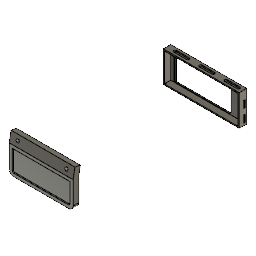
GPU mount (Autodesk Fusion 360 design; units mm, degrees)
Autodesk Fusion 360 part; units mm, degrees
sketch "imac body" plane through (0, 0, 0) normal (0, 0, 1) x (1, 0, 0)
  line L0 (-150, -55) -> (150, -55)
  line L1 (150, -55) -> (150, 150)
  line L2 (20, 280) -> (-20, 280)
  line L3 (-150, 150) -> (-150, -55)
  line L4 (0, 280) -> (0, -55) construction
  line L5 (0, 0) -> (150, 0) construction
  arc A0 (-20, 280) -> (-150, 150) centre (-20, 150) ccw
  arc A1 (150, 150) -> (20, 280) centre (20, 150) ccw
  line L6 (150, 0) -> (-150, 0)
  line L7 (-93.6888, 60) -> (93.6888, 60)
  line L8 (93.6888, 60) -> (93.6888, 40)
  line L9 (93.6888, 40) -> (-93.6888, 40)
  line L10 (-93.6888, 40) -> (-93.6888, 60)
  dimension "d1" = 280
  dimension "d2" = 55
  dimension "d3" = 300
  dimension "d4" = 130
  dimension "d7" = 40
  dimension "d8" = 20
  constraint horizontal L0
  constraint vertical L1
  constraint horizontal L2
  constraint vertical L3
  constraint midpoint L0 L4.end
  constraint coincident L5.start L4
  constraint coincident L5.start origin
  constraint coincident L1 L5.end
  constraint perpendicular L1 L5
  constraint coincident L2 L4.start
  constraint tangent L2 A0
  constraint tangent L3 A0
  constraint tangent L1 A1
  constraint tangent L2 A1
  constraint equal A0 A1
  constraint coincident L3 L6.end
  constraint perpendicular L3 L6
  constraint horizontal L7
  constraint vertical L8
  constraint horizontal L9
  constraint vertical L10
  measures "d1" distance of L2 L5
  measures "d2" distance of L0 L5 L3.end
  measures "d3" distance of L1 L3
  measures "d4" radius of A0
  measures "d7" distance of L6 L9
  measures "d8" distance of L7 L9
  measures "d62" distance of L0.start
  measures "d83" distance of L0.start
extrude "Extrude1" add sketch "imac body" along normal blind 2 contours L1 L2 L3 A0 A1 L6 | L7 L8 L9 L10 makes body 1
extrude "Extrude2" add sketch "imac body" against normal blind 5 contours L7 L8 L9 L10 bodies 1
ref_plane "WorkPlane1" through (0, 0, 0) normal (0, 0.173648, 0.984808) x (-1, 0, 0)
sketch "imac body bend" plane through (0, 0, 0) normal (0, 0.173648, 0.984808) x (-1, 0, 0)
  line L0 (-150, 0) -> (150, 0)
  line L1 (-150, 0) -> (150, 0)
  line L2 (150, 0) -> (150, 55)
  line L3 (150, 55) -> (-150, 55)
  line L4 (-150, 55) -> (-150, 0)
  dimension "d32" = 55
  constraint horizontal L1
  constraint vertical L2
  constraint horizontal L3
  constraint vertical L4
  constraint coincident L0.start L1.start
  measures "d32" distance of L0.start L3.end
extrude "Extrude3" add sketch "imac body bend" along normal blind 2 bodies 1
sketch "gpu body" plane through (0, 0, 0) normal (0, 0, 1) x (1, 0, 0)
  line L0 (47.5, 132.5) -> (-47.5, 132.5)
  line L1 (-47.5, 132.5) -> (-47.5, -132.5)
  line L2 (-47.5, -132.5) -> (47.5, -132.5)
  line L3 (47.5, -132.5) -> (47.5, 132.5)
  line L4 (47.5, 132.5) -> (-47.5, -132.5) construction
  line L5 (-47.5, 132.5) -> (47.5, -132.5) construction
  line L6 (0, 132.5) -> (0, -132.5) construction
  circle A0 centre (0, -59.5) radius 32.5
  line L7 (-47.5, 132.5) -> (47.5, 132.5)
  line L8 (47.5, 132.5) -> (47.5, 136.5)
  line L9 (47.5, 136.5) -> (-47.5, 136.5)
  line L10 (-47.5, 136.5) -> (-47.5, 132.5)
  line L11 (-44.5, 136.5) -> (-42.5, 136.5)
  line L12 (-42.5, 136.5) -> (-42.5, 148.5)
  line L13 (-42.5, 148.5) -> (-44.5, 148.5)
  line L14 (-44.5, 148.5) -> (-44.5, 136.5)
  line L15 (-44.5, 136.5) -> (-44.5, 132.5)
  dimension "d14" = 265
  dimension "d15" = 95
  dimension "d18" = 65
  dimension "d19" = 73
  dimension "d20" = 4
  dimension "d21" = 2
  dimension "d22" = 12
  dimension "d23" = 3
  constraint perpendicular L0 L1
  constraint parallel L0 L2
  constraint parallel L1 L3
  constraint horizontal L0
  constraint coincident L4 origin
  constraint coincident L5 origin
  constraint midpoint L0 L6.start
  constraint midpoint L2 L6.end
  constraint coincident L6 A0.centre
  constraint horizontal L7
  constraint vertical L8
  constraint horizontal L9
  constraint vertical L10
  constraint horizontal L11
  constraint vertical L12
  constraint horizontal L13
  constraint vertical L14
  constraint coincident L9 L11.start
  constraint coincident L7 L15.end
  constraint perpendicular L7 L15
  measures "d14" distance of L0.end L1.end
  measures "d15" distance of L1.end L2.end
  measures "d18" diameter of A0
  measures "d19" distance of L6.end A0.centre
  measures "d20" distance of L7 L9
  measures "d21" distance of L12 L14
  measures "d22" distance of L9 L13
  measures "d23" distance of L9.end L11.start
extrude "Extrude4" add sketch "gpu body" against normal blind 37 separate body contours L0 L1 L2 L3 L7 | L0 L7 L8 L9 L11 L15 | L9 L11 L12 L13 L14 | A0 makes body 2
extrude "Extrude5" cut sketch "gpu body" along normal blind 3 from surface at -37 contours A0 bodies 2
sketch "gpu psu connector" plane through (-47.5, 0, 0) normal (-1, 0, 0) x (0, -1, 0)
  line L0 (132.5, 0) -> (-132.5, 0)
  line L1 (-132.5, 0) -> (-132.5, -37)
  line L2 (-132.5, -37) -> (132.5, -37)
  line L3 (132.5, -37) -> (132.5, 0)
  line L4 (122.5, 0) -> (80.5, 0)
  line L5 (80.5, 0) -> (80.5, -20)
  line L6 (80.5, -20) -> (122.5, -20)
  line L7 (122.5, -20) -> (122.5, 0)
  dimension "d27" = 10
  dimension "d28" = 42
  dimension "d29" = 20
  constraint horizontal L4
  constraint vertical L5
  constraint horizontal L6
  constraint vertical L7
  constraint coincident L0 L4.start
  measures "d27" distance of L3 L7
  measures "d28" distance of L5 L7
  measures "d29" distance of L4 L6
extrude "Extrude6" add sketch "gpu psu connector" along normal blind 10 contours L0 L4 L5 L6 L7 bodies 2
move_body "Move5" bodies 2 to x (1, 0, 0) y (0, 1, 0) z (0, 0, 1) at (0, 63, -10)
sketch "gpu front connector" plane through (47.5, 0, 0) normal (1, 0, 0) x (0, 1, 0)
  line L0 (199.5, -47) -> (199.5, -10)
  line L1 (199.5, -10) -> (-69.5, -10)
  line L2 (-69.5, -10) -> (-69.5, -47)
  line L3 (197.0366, -14.7221) -> (198.5366, -14.7221)
  line L4 (198.5366, -14.7221) -> (198.5366, -24.7221)
  line L5 (198.5366, -24.7221) -> (197.0366, -24.7221)
  line L6 (197.0366, -24.7221) -> (197.0366, -14.7221)
  line L7 (197.0366, -34.7221) -> (198.5366, -34.7221)
  line L8 (198.5366, -34.7221) -> (198.5366, -44.7221)
  line L9 (198.5366, -44.7221) -> (197.0366, -44.7221)
  line L10 (197.0366, -44.7221) -> (197.0366, -34.7221)
  circle A0 centre (203.3196, -12.8419) radius 2.25
  circle A1 centre (203.3196, -28.3419) radius 2.25
  line L11 (-69.5, -47) -> (199.5, -47)
  line L12 (199.5, -47) -> (196.0366, -47)
  line L13 (196.0366, -47) -> (196.0366, -10)
  line L14 (196.0366, -10) -> (199.5, -10)
  line L15 (199.5, -10) -> (199.5, -47)
  line L16 (199.0366, -25.2221) -> (196.5366, -25.2221)
  line L17 (196.5366, -25.2221) -> (196.5366, -14.2221)
  line L18 (196.5366, -14.2221) -> (199.0366, -14.2221)
  line L19 (199.0366, -14.2221) -> (199.0366, -25.2221)
  line L20 (199.0366, -45.2221) -> (196.5366, -45.2221)
  line L21 (196.5366, -45.2221) -> (196.5366, -34.2221)
  line L22 (196.5366, -34.2221) -> (199.0366, -34.2221)
  line L23 (199.0366, -34.2221) -> (199.0366, -45.2221)
  dimension "d61" = 1.5
  dimension "d62" = 10
  dimension "d63" = 1.5
  dimension "d64" = 10
  dimension "d65" = 10
  dimension "d69" = 4.5
  dimension "d70" = 4.5
  dimension "d71" = 15.5
  dimension "d83" = 1
  dimension "d84" = -0.5
  dimension "d85" = -0.5
  constraint horizontal L3
  constraint vertical L4
  constraint horizontal L5
  constraint vertical L6
  constraint horizontal L7
  constraint vertical L8
  constraint horizontal L9
  constraint vertical L10
  constraint horizontal L12
  constraint vertical L13
  constraint horizontal L14
  constraint vertical L15
  constraint coincident L1 L13.end
  constraint coincident L0.start L11.end
  constraint collinear L17 L21
  measures "d61" distance of L3.start L3.end
  measures "d62" distance of L3.start L5.end
  measures "d63" distance of L7.start L7.end
  measures "d64" distance of L7.start L9.end
  measures "d65" distance of L5 L7
  measures "d69" diameter of A0
  measures "d70" diameter of A1
  measures "d71" distance of A0.centre A1.centre
  measures "d83" distance of L6 L13
extrude "Extrude13" add sketch "gpu front connector" along normal blind 29 contours L3 L4 L5 L6 | L7 L8 L9 L10 bodies 2
extrude "Extrude14" cut sketch "gpu front connector" against normal blind 100 contours A0 | A1 bodies 2
fillet "Fillet2" radius 4 2 edges at (-47.5, 63, -47) (47.5, 65, -47) on bodies 2
sketch "gpu front mount" plane through (0, 199.5, 0) normal (0, 1, 0) x (-1, 0, 0)
  arc A0 (-47.5, -43) -> (-43.5, -47) centre (-43.5, -43) ccw
  line L0 (-43.5, -47) -> (42.5, -47)
  line L1 (42.5, -47) -> (42.5, -10)
  line L2 (42.5, -10) -> (-47.5, -10)
  line L3 (-47.5, -10) -> (-47.5, -43)
  line L4 (44.5, -10) -> (44.5, -46.873)
  line L5 (47.5, -10) -> (47.5, -43)
  line L6 (-47.5, -14.7221) -> (-76.5, -14.7221)
  line L7 (-76.5, -24.7221) -> (-76.5, -14.7221)
  line L8 (-47.5, -24.7221) -> (-76.5, -24.7221)
  line L9 (-47.5, -34.7221) -> (-76.5, -34.7221)
  line L10 (-76.5, -44.7221) -> (-76.5, -34.7221)
  line L11 (-76.5, -44.7221) -> (-47.1103, -44.7221)
  line L12 (-43.5, -49) -> (42.5, -49) construction
  line L13 (-67.5, -49) -> (50.5, -49)
  line L14 (50.5, -49) -> (50.5, 0)
  line L15 (-67.5, 0) -> (-67.5, -49)
  arc A1 (-46.5, -43) -> (-43.5, -46) centre (-43.5, -43) ccw
  line L16 (-43.5, -46) -> (41.5, -46)
  line L17 (41.5, -46) -> (41.5, -11)
  line L18 (41.5, -11) -> (-46.5, -11)
  line L19 (-46.5, -11) -> (-46.5, -43)
  line L20 (150, 0) -> (20, 0)
  line L21 (-20, 0) -> (20, 0)
  line L22 (-20, 0) -> (-150, 0)
  line L23 (-43.5, -47) -> (-67.5, -47)
  arc A2 (43.5, -47) -> (44.5, -46.873) centre (43.5, -43) ccw
  line L24 (44.5, -46.873) -> (44.5, -10)
  line L25 (44.5, -10) -> (42.5, -10)
  line L26 (42.5, -10) -> (42.5, -47)
  line L27 (42.5, -47) -> (43.5, -47)
  line L28 (43.5, -47) -> (50.5, -47)
  line L29 (48.5, 0) -> (48.5, -47)
  dimension "d75" = 2
  dimension "d76" = -1
  dimension "d81" = 6
  dimension "d82" = 112
  dimension "d99" = 2
  constraint horizontal L13
  constraint vertical L14
  constraint vertical L15
  constraint coincident L12.start L13
  constraint coincident L15.start L22
  constraint coincident L14.end L20
  constraint coincident A0.end L0.start
  constraint tangent A0 L23
  constraint coincident L15 L23.end
  constraint coincident A2.start L27.end
  constraint coincident L14 L28.end
  constraint tangent A2 L28
  constraint coincident L20 L29.start
  constraint coincident L28 L29.end
  constraint perpendicular L28 L29
  measures "d81" distance of L4 L14
  measures "d82" distance of L4 L15
  measures "d99" distance of L14 L29
extrude "Extrude15" add sketch "gpu front mount" along normal blind 2 separate body contours A0 L0 L1 L2 L3 L26 | A0 L3 L9 L11 L15 | A0 L11 L15 L23 | L3 L8 L9 L15 | L0 L13 L14 L15 L23 L27 L28 | L3 L6 L8 L15 | L2 L3 L4 L6 L15 L20 L21 L22 A2 L24 L25 L28 L29 | L14 L20 L28 L29 makes body 3
extrude "Extrude17" add sketch "gpu front mount" against normal blind 10 contours L0 L13 L14 L15 L23 L27 L28 | L14 L20 L28 L29 bodies 3
sketch "gpu front mount side" plane through (47.5, 0, 0) normal (1, 0, 0) x (0, 1, 0)
  line L0 (198.5366, -43) -> (199.5, -43)
  line L1 (199.5, -10) -> (-69.5, -10)
  line L2 (-69.5, -10) -> (-69.5, -43)
  line L3 (-69.5, -43) -> (197.0366, -43)
  line L4 (197.0366, -43) -> (197.0366, -34.7221)
  line L5 (197.0366, -34.7221) -> (198.5366, -34.7221)
  line L6 (198.5366, -34.7221) -> (198.5366, -43)
  line L7 (197.0366, -24.7221) -> (197.0366, -14.7221)
  line L8 (197.0366, -14.7221) -> (198.5366, -14.7221)
  line L9 (198.5366, -14.7221) -> (198.5366, -24.7221)
  line L10 (198.5366, -24.7221) -> (197.0366, -24.7221)
  line L11 (196.5366, -34.2221) -> (199.0366, -34.2221)
  line L12 (196.5366, -45.2221) -> (196.5366, -34.2221)
  line L13 (199.0366, -34.2221) -> (199.0366, -45.2221)
  line L14 (199.0366, -45.2221) -> (196.5366, -45.2221)
  line L15 (199.0366, -25.2221) -> (196.5366, -25.2221)
  line L16 (196.5366, -25.2221) -> (196.5366, -14.2221)
  line L17 (199.0366, -14.2221) -> (199.0366, -25.2221)
  line L18 (196.5366, -14.2221) -> (199.0366, -14.2221)
  line L19 (199.5, 0) -> (199.5, -47)
  line L20 (189.5, -49) -> (201.5, -49)
  line L21 (201.5, -49) -> (201.5, 0)
  line L22 (201.5, 0) -> (199.5, 0)
  line L23 (199.5, -47) -> (189.5, -47)
  line L24 (189.5, -47) -> (189.5, 0)
  line L25 (189.5, 0) -> (199.5, 0)
  line L26 (199.5, 0) -> (199.5, -47)
  line L27 (199.5, -47) -> (189.5, -47)
  line L28 (189.5, -47) -> (189.5, -49)
  line L29 (199.5, -43) -> (199.5, -10)
  dimension "d86" = 10
  constraint horizontal L23
  constraint vertical L24
  constraint horizontal L25
  constraint vertical L26
  constraint coincident L19.end L23.start
  constraint coincident L19.start L22.end
  measures "d86" distance of L19.end L23.end
extrude "Extrude16" add sketch "gpu front mount side" along normal blind 2 from surface at 20 contours L0 L1 L3 L11 L12 L13 L19 L24 L26 L29 | L0 L3 L12 L13 L14 L19 L23 L24 L26 L27 | L19 L20 L21 L22 L23 L26 L27 L28 L29 | L1 L19 L24 L25 L26 bodies 3
sketch "gpu front mount top" plane through (0, 0, 0) normal (0, 0, -1) x (1, 0, 0)
  line L0 (93.6888, -40) -> (93.6888, -60)
  line L1 (93.6888, -60) -> (-93.6888, -60)
  line L2 (-93.6888, -60) -> (-93.6888, -40)
  line L3 (-93.6888, -40) -> (93.6888, -40)
  arc A0 (20, -280) -> (150, -150) centre (20, -150) ccw
  line L4 (150, -150) -> (150, 0)
  line L5 (150, 0) -> (-150, 0)
  line L6 (-150, 0) -> (-150, -150)
  arc A1 (-150, -150) -> (-20, -280) centre (-20, -150) ccw
  line L7 (-20, -280) -> (20, -280)
  line L8 (-50.5, -189.5) -> (-50.5, -201.5)
  line L9 (-50.5, -201.5) -> (69.5, -201.5)
  line L10 (69.5, -201.5) -> (69.5, -189.5)
  line L11 (69.5, -189.5) -> (-50.5, -189.5)
  circle A2 centre (-37.581, -195.5) radius 2.25
  circle A3 centre (-17.581, -195.5) radius 2.25
  circle A4 centre (2.419, -195.5) radius 2.25
  circle A5 centre (22.419, -195.5) radius 2.25
  circle A6 centre (42.419, -195.5) radius 2.25
  circle A7 centre (62.419, -195.5) radius 2.25
  line L12 (-37.581, -193.25) -> (-17.581, -193.25)
  line L13 (-17.581, -197.75) -> (-37.581, -197.75)
  line L14 (2.419, -193.25) -> (22.419, -193.25)
  line L15 (22.419, -197.75) -> (2.419, -197.75)
  line L16 (42.419, -193.25) -> (62.419, -193.25)
  line L17 (62.419, -197.75) -> (42.419, -197.75)
  dimension "d92" = 4.5
  dimension "d95" = 100
  dimension "d96" = 0
  constraint coincident A2 L12.start
  constraint coincident A3 L12.end
  constraint tangent A3 L12
  constraint perpendicular L8 L12
  constraint coincident A3 L13.start
  constraint coincident A2 L13.end
  constraint tangent A2 L13
  constraint perpendicular L8 L13
  constraint coincident A4 L14.start
  constraint coincident A5 L14.end
  constraint tangent A5 L14
  constraint parallel L13 L14
  constraint coincident A5 L15.start
  constraint coincident A4 L15.end
  constraint tangent A4 L15
  constraint parallel L14 L15
  constraint coincident A6 L16.start
  constraint coincident A7 L16.end
  constraint tangent A7 L16
  constraint parallel L15 L16
  constraint coincident A7 L17.start
  constraint coincident A6 L17.end
  constraint tangent A6 L17
  constraint parallel L16 L17
  measures "d92" diameter of A2
extrude "Extrude18" add sketch "gpu front mount top" along normal blind 2 contours L8 L9 L10 L11 bodies 3
sketch "gpu back back side" plane through (0, -69.5, 0) normal (0, -1, 0) x (1, 0, 0)
  arc A0 (43.5, -47) -> (47.5, -43) centre (43.5, -43) ccw
  line L0 (47.5, -43) -> (47.5, -10)
  line L1 (47.5, -10) -> (-47.5, -10)
  line L2 (-47.5, -10) -> (-47.5, -43)
  arc A1 (-47.5, -43) -> (-43.5, -47) centre (-43.5, -43) ccw
  line L3 (-43.5, -47) -> (43.5, -47)
  arc A2 (-48.5, -43) -> (-43.5, -48) centre (-43.5, -43) ccw
  line L4 (-43.5, -48) -> (43.5, -48)
  arc A3 (43.5, -48) -> (48.5, -43) centre (43.5, -43) ccw
  line L5 (48.5, -43) -> (48.5, -9)
  line L6 (48.5, -9) -> (-48.5, -9)
  line L7 (-48.5, -9) -> (-48.5, -43)
  arc A4 (-50.5, -43) -> (-43.5, -50) centre (-43.5, -43) ccw
  line L8 (-43.5, -50) -> (43.5, -50)
  arc A5 (43.5, -50) -> (50.5, -43) centre (43.5, -43) ccw
  line L9 (50.5, -43) -> (50.5, -7)
  line L10 (50.5, -7) -> (-50.5, -7) construction
  line L11 (-50.5, -7) -> (-50.5, -43)
  line L12 (-50.5, -7) -> (50.5, -7)
  line L13 (50.5, -7) -> (50.5, -6.9921)
  line L14 (50.5, -6.9921) -> (-50.5, -6.9921)
  line L15 (-50.5, -6.9921) -> (-50.5, -7)
  line L16 (-48.5, -9) -> (-48.5, -7)
  line L17 (48.5, -9) -> (48.5, -7)
  arc A6 (-45.5, -43) -> (-43.5, -45) centre (-43.5, -43) ccw
  line L18 (-43.5, -45) -> (43.5, -45)
  arc A7 (43.5, -45) -> (45.5, -43) centre (43.5, -43) ccw
  line L19 (45.5, -43) -> (45.5, -12)
  line L20 (45.5, -12) -> (-45.5, -12)
  line L21 (-45.5, -12) -> (-45.5, -43)
  dimension "d100" = 1
  dimension "d101" = 3
  dimension "d103" = -2
  dimension "d126" = 2.0079
  constraint horizontal L12
  constraint vertical L13
  constraint horizontal L14
  constraint vertical L15
  constraint coincident L12 L16.end
  constraint perpendicular L12 L16
  constraint coincident L10 L17.end
  constraint perpendicular L10 L17
  measures "d126" distance of L6 L14
extrude "Extrude19" add sketch "gpu back back side" along normal blind 2 separate body contours A0 L0 L1 L2 A1 L3 | A2 L4 A3 L5 L6 L7 | A2 L4 A3 L5 L7 A4 L8 A5 L9 L11 L12 L16 L17 | L6 L12 L16 L17 | L12 L13 L14 L15 makes body 4
extrude "Extrude20" add sketch "gpu back back side" against normal blind 7 contours A0 L0 L1 L2 A1 L3 | A2 L4 A3 L5 L6 L7 | A2 L4 A3 L5 L7 A4 L8 A5 L9 L11 L12 L16 L17 | L6 L12 L16 L17 | L12 L13 L14 L15 | A6 L18 A7 L19 L20 L21 bodies 4
sketch "gpu back top " plane through (0, 0, 0) normal (0, -0.173648, -0.984808) x (1, 0, 0)
  line L0 (150, 0) -> (150, 55)
  line L1 (150, 55) -> (-150, 55) construction
  line L2 (-150, 55) -> (-150, 0)
  line L3 (-150, 0) -> (150, 0)
  line L4 (-50.5, 60.3363) -> (-50.5, 69.1996) construction
  line L5 (-50.5, 69.1996) -> (50.5, 69.1996) construction
  line L6 (50.5, 69.1996) -> (50.5, 60.3363) construction
  line L7 (50.5, 60.3363) -> (-50.5, 60.3363) construction
  line L8 (-50.5, 55) -> (50.5, 55)
  line L9 (50.5, 55) -> (50.5, 35)
  line L10 (50.5, 35) -> (-50.5, 35)
  line L11 (-50.5, 35) -> (-50.5, 55)
  line L12 (50.5, 55) -> (50.5, 58)
  line L13 (50.5, 58) -> (-50.5, 58)
  line L14 (-50.5, 58) -> (-50.5, 55)
  circle A0 centre (-43.5699, 45) radius 2.25
  circle A1 centre (-26.5699, 45) radius 2.25
  circle A2 centre (-9.5699, 45) radius 2.25
  circle A3 centre (7.4301, 45) radius 2.25
  circle A4 centre (24.4301, 45) radius 2.25
  circle A5 centre (41.4301, 45) radius 2.25
  line L15 (-43.5699, 47.25) -> (-26.5699, 47.25)
  line L16 (-26.5699, 42.75) -> (-43.5699, 42.75)
  line L17 (-9.5699, 42.75) -> (7.4301, 42.75)
  line L18 (7.4301, 47.25) -> (-9.5699, 47.25)
  line L19 (24.4301, 47.25) -> (41.4301, 47.25)
  line L20 (41.4301, 42.75) -> (24.4301, 42.75)
  line L21 (-43.5699, 45) -> (41.4301, 45) construction
  dimension "d108" = 20
  dimension "d109" = 3
  dimension "d115" = 4.5
  dimension "d118" = 85
  dimension "d119" = 0
  dimension "d125" = 10
  constraint horizontal L8
  constraint vertical L9
  constraint horizontal L10
  constraint vertical L11
  constraint coincident L1 L8.start
  constraint vertical L12
  constraint horizontal L13
  constraint vertical L14
  constraint coincident A0 L15.start
  constraint coincident A1 L15.end
  constraint tangent A1 L15
  constraint parallel L8 L15
  constraint coincident A1 L16.start
  constraint coincident A0 L16.end
  constraint tangent A0 L16
  constraint parallel L8 L16
  constraint coincident A2 L17.start
  constraint coincident A3 L17.end
  constraint tangent A3 L17
  constraint parallel L16 L17
  constraint coincident A3 L18.start
  constraint coincident A2 L18.end
  constraint tangent A2 L18
  constraint parallel L17 L18
  constraint coincident A4 L19.start
  constraint coincident A5 L19.end
  constraint tangent A5 L19
  constraint parallel L18 L19
  constraint coincident A5 L20.start
  constraint coincident A4 L20.end
  constraint tangent A4 L20
  constraint parallel L19 L20
  constraint coincident A0.centre L21.start
  constraint coincident A5.centre L21.end
  constraint coincident A3.centre A4.centre
  constraint coincident A2.centre A3.centre
  constraint coincident A1.centre A2.centre
  measures "d108" distance of L8.start L10.end
  measures "d109" distance of L8.start L13.end
  measures "d115" diameter of A0
  measures "d125" distance of L8 L21
move_body "Move7" bodies 4 to x (1, 0, 0) y (0, 1, 0) z (0, 0, 1) at (0, 18, 0)
sketch "Sketch16" plane through (0, 0, 0) normal (0, -0.173648, -0.984808) x (1, 0, 0)
  line L0 (150, 0) -> (150, 55)
  line L1 (150, 55) -> (-150, 55)
  line L2 (-150, 55) -> (-150, 0)
  line L3 (-150, 0) -> (150, 0)
  line L4 (-50.5, 42.6098) -> (-50.5, 51.473)
  line L5 (-50.5, 51.473) -> (50.5, 51.473)
  line L6 (50.5, 51.473) -> (50.5, 42.6098)
  line L7 (50.5, 42.6098) -> (-50.5, 42.6098)
loft "Loft3" add profiles "Sketch16" section 1 face at (-16.8333, -50.5, -6.9921) section 2 contours L4 L5 L6 L7 on bodies 4 bodies 4
sketch "Sketch17" plane through (0, -50.691, 8.9382) normal (0, -0.984808, 0.173648) x (1, 0, 0)
  line L0 (-50.5, -16.1761) -> (50.5, -16.1761)
  line L1 (50.5, -16.1761) -> (50.5, 0)
  line L2 (50.5, 0) -> (-50.5, 0)
  line L3 (-50.5, 0) -> (-50.5, -16.1761)
  line L4 (-50.5, -8.0881) -> (50.5, -8.0881) construction
  circle A0 centre (-38.5, -8.0881) radius 2.5
  circle A1 centre (38.5, -8.0881) radius 2.6612
  dimension "d127" = 5
  dimension "d128" = 77
  dimension "d129" = 38.5
  constraint midpoint L3 L4.start
  constraint midpoint L1 L4.end
  constraint coincident L4 A0.centre
  constraint coincident L4 A1.centre
  measures "d127" diameter of A0
  measures "d128" distance of A0.centre A1.centre
  measures "d129" horizontal distance of origin A0.centre
extrude "Extrude24" cut sketch "Sketch17" against normal blind 20 contours A0 | A1 bodies 4
extrude "Extrude21" [rolled back] profile offset -3 along distance -2 taper angle 0
extrude "Extrude22" [rolled back] along distance -5 taper angle 0
loft "Loft2" [rolled back]
extrude "Extrude23" [rolled back] along distance 2 taper angle 0
fillet "Fillet3" [rolled back] radius 426 radius 3 radius 4.5
hidden bodies 1 2
equation "d129 = ( 77 / 2 ) * 1 mm"
named bodies: "iMac body", "INNO3D 2070 SUPER JET", "Front bracket", "Back bracket"
